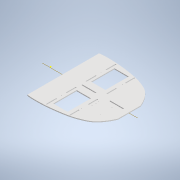
# Autodesk Inventor part: head_1
Saved by Autodesk Inventor 2020 (Build 240168000, 168)
## iProperties
Created: 2022-02-10
Part Number: head_1
Material: Типовые
Document SubType Name: Modeling
Designer: HP
Density: 1 g/cm^3
Appearance: По умолчанию
Mass: 318.083 g
Surface Area: 1630.63 cm^2
Volume: 318.083 cm^3
Author: HP
Autodesk Inventor part; units mm, degrees
ref_plane "YZ Plane" through (0, 0, 0) normal (1, 0, 0) x (0, 1, 0)
ref_plane "XZ Plane" through (0, 0, 0) normal (0, 1, 0) x (-1, 0, 0)
ref_plane "XY Plane" through (0, 0, 0) normal (0, 0, 1) x (1, 0, 0)
sketch "Эскиз1" plane through (0, 0, 0) normal (0, 1, 0) x (-1, 0, 0)
  line L0 (0, 0) -> (-339.5216, 0)
  line L1 (-129.0273, 2.0017) -> (-133.0273, 2.0017) construction
  line L2 (-133.0273, 20.9197) -> (-133.0273, 2.0017) construction
  line L3 (-133.0273, 20.9197) -> (-129.0273, 20.9197) construction
  line L4 (-129.0273, 20.9197) -> (-129.0273, 2.0017) construction
  line L5 (-129.0273, 2.0017) -> (-129.0273, -5.9794)
  line L6 (-10.1099, 0) -> (-40.1099, 0)
  line L7 (-53.7435, -154.1362) -> (-65.8717, -156.1972) construction
  line L8 (-65.8717, -156.1972) -> (-85.3727, -156.99) construction
  line L9 (-85.3727, -156.99) -> (-121.6794, -156.0387) construction
  line L10 (-121.6794, -156.0387) -> (-146.4123, -154.1362) construction
  line L11 (-146.4123, -154.1362) -> (-185.0972, -149.2213) construction
  line L12 (-185.0972, -149.2213) -> (-220.9282, -142.8795) construction
  line L13 (-220.9282, -142.8795) -> (-240.4292, -137.6475) construction
  line L14 (-240.4292, -137.6475) -> (-274.3577, -124.964) construction
  line L15 (-274.3577, -124.964) -> (-292.7488, -114.0244) construction
  line L16 (-292.7488, -114.0244) -> (-307.3349, -99.5969) construction
  line L17 (-307.3349, -99.5969) -> (-319.3843, -84.5352) construction
  line L18 (-319.3843, -84.5352) -> (-329.3726, -68.2051) construction
  line L19 (-329.3726, -68.2051) -> (-336.6657, -52.6677) construction
  line L20 (-336.6657, -52.6677) -> (-338.102, -47.8439) construction
  spline S0 degree 4 poles (-53.7435, -154.1362) (-65.8717, -156.1972) (-85.3727, -156.99) (-121.6794, -156.0387) (-146.4123, -154.1362) (-185.0972, -149.2213) (-220.9282, -142.8795) (-240.4292, -137.6475) (-274.3577, -124.964) (-292.7488, -114.0244) (-307.3349, -99.5969) (-319.3843, -84.5352) (-329.3726, -68.2051) (-336.6657, -52.6677) (-338.102, -47.8439) knots 1 1 1 1 1 2 3 4 5 6 7 8 9 10 11 12 12 12 12 12
  line L21 (-338.102, -47.8439) -> (-338.102, 0)
  line L22 (-53.7435, 154.1362) -> (-65.8717, 156.1972) construction
  line L23 (-65.8717, 156.1972) -> (-85.3727, 156.99) construction
  line L24 (-85.3727, 156.99) -> (-121.6794, 156.0387) construction
  line L25 (-121.6794, 156.0387) -> (-146.4123, 154.1362) construction
  line L26 (-146.4123, 154.1362) -> (-185.0972, 149.2213) construction
  line L27 (-185.0972, 149.2213) -> (-220.9282, 142.8795) construction
  line L28 (-220.9282, 142.8795) -> (-240.4292, 137.6475) construction
  line L29 (-240.4292, 137.6475) -> (-274.3577, 124.964) construction
  line L30 (-274.3577, 124.964) -> (-292.7488, 114.0244) construction
  line L31 (-292.7488, 114.0244) -> (-307.3349, 99.5969) construction
  line L32 (-307.3349, 99.5969) -> (-319.3843, 84.5352) construction
  line L33 (-319.3843, 84.5352) -> (-329.3726, 68.2051) construction
  line L34 (-329.3726, 68.2051) -> (-336.6657, 52.6677) construction
  line L35 (-336.6657, 52.6677) -> (-338.102, 47.8439) construction
  spline S1 degree 4 poles (-53.7435, 154.1362) (-65.8717, 156.1972) (-85.3727, 156.99) (-121.6794, 156.0387) (-146.4123, 154.1362) (-185.0972, 149.2213) (-220.9282, 142.8795) (-240.4292, 137.6475) (-274.3577, 124.964) (-292.7488, 114.0244) (-307.3349, 99.5969) (-319.3843, 84.5352) (-329.3726, 68.2051) (-336.6657, 52.6677) (-338.102, 47.8439) knots 1 1 1 1 1 2 3 4 5 6 7 8 9 10 11 12 12 12 12 12
  line L36 (-338.102, 47.8439) -> (-338.102, 0)
  line L37 (-144.7435, 0) -> (-53.7435, 0)
  line L38 (-53.7435, 0) -> (-53.7435, -154.1362)
  line L39 (-53.7435, 154.1362) -> (-65.8717, 156.1972) construction
  line L40 (-65.8717, 156.1972) -> (-85.3727, 156.99) construction
  line L41 (-85.3727, 156.99) -> (-121.6794, 156.0387) construction
  line L42 (-121.6794, 156.0387) -> (-146.4123, 154.1362) construction
  line L43 (-146.4123, 154.1362) -> (-185.0972, 149.2213) construction
  line L44 (-185.0972, 149.2213) -> (-220.9282, 142.8795) construction
  line L45 (-220.9282, 142.8795) -> (-240.4292, 137.6475) construction
  line L46 (-240.4292, 137.6475) -> (-274.3577, 124.964) construction
  line L47 (-274.3577, 124.964) -> (-292.7488, 114.0244) construction
  line L48 (-292.7488, 114.0244) -> (-307.3349, 99.5969) construction
  line L49 (-307.3349, 99.5969) -> (-319.3843, 84.5352) construction
  line L50 (-319.3843, 84.5352) -> (-329.3726, 68.2051) construction
  line L51 (-329.3726, 68.2051) -> (-336.6657, 52.6677) construction
  line L52 (-336.6657, 52.6677) -> (-338.102, 47.8439) construction
  spline S2 degree 4 poles (-53.7435, 154.1362) (-65.8717, 156.1972) (-85.3727, 156.99) (-121.6794, 156.0387) (-146.4123, 154.1362) (-185.0972, 149.2213) (-220.9282, 142.8795) (-240.4292, 137.6475) (-274.3577, 124.964) (-292.7488, 114.0244) (-307.3349, 99.5969) (-319.3843, 84.5352) (-329.3726, 68.2051) (-336.6657, 52.6677) (-338.102, 47.8439) knots 1 1 1 1 1 2 3 4 5 6 7 8 9 10 11 12 12 12 12 12
  line L53 (-338.102, 47.8439) -> (-338.102, 0)
  line L54 (-53.7435, 0) -> (-53.7435, 154.1362)
  point P0 (-144.7435, 57.7778)
  dimension "d42" = 30
  constraints: 18 end point, 15 symmetric about line, 5 point on line, 2 perpendicular, 1 horizontal, 1 vertical, 9 other
  measures "d42" distance of L6.start L6.end
extrude "Выдавливание1" add sketch "Эскиз1" along normal blind 4
sketch "Эскиз2" plane through (0, 0, 0) normal (0, -1, 0) x (1, 0, 0)
  line L0 (224, 59.917) -> (220, 59.917) projected
  line L1 (220, 59.917) -> (220, 19.9723) projected
  line L2 (220, 19.9723) -> (224, 19.9723) projected
  line L3 (224, 19.9723) -> (224, 59.917) projected
  line L4 (220, 99.8616) -> (224, 99.8616) projected
  line L5 (224, 99.8616) -> (224, 139.8063) projected
  line L6 (224, 139.8063) -> (220, 139.8063) projected
  line L7 (220, 139.8063) -> (220, 99.8616) projected
  line L8 (224, -19.9723) -> (220, -19.9723) projected
  line L9 (220, -19.9723) -> (220, -59.917) projected
  line L10 (220, -59.917) -> (224, -59.917) projected
  line L11 (224, -59.917) -> (224, -19.9723) projected
  line L12 (224, -99.8616) -> (220, -99.8616) projected
  line L13 (220, -99.8616) -> (220, -139.8063) projected
  line L14 (220, -139.8063) -> (224, -139.8063) projected
  line L15 (224, -139.8063) -> (224, -99.8616) projected
  line L16 (220, 19.9723) -> (219.5, 19.9723)
  line L17 (219.5, 19.9723) -> (219.5, 59.917)
  line L18 (219.5, 59.917) -> (220, 59.917)
  line L19 (224, 59.917) -> (224.5, 59.917)
  line L20 (224.5, 59.917) -> (224.5, 19.9723)
  line L21 (224.5, 19.9723) -> (224, 19.9723)
  line L22 (220, 99.8616) -> (219.5, 99.8616)
  line L23 (219.5, 99.8616) -> (219.5, 139.8063)
  line L24 (219.5, 139.8063) -> (220, 139.8063)
  line L25 (224, 99.8616) -> (224.5, 99.8616)
  line L26 (224.5, 99.8616) -> (224.5, 139.8063)
  line L27 (224.5, 139.8063) -> (224, 139.8063)
  line L28 (197.5179, 0) -> (240.56, 0)
  line L29 (224, -59.917) -> (220, -59.917)
  line L30 (220, -59.917) -> (220, -19.9723)
  line L31 (220, -19.9723) -> (224, -19.9723)
  line L32 (224, -19.9723) -> (224, -59.917)
  line L33 (220, -99.8616) -> (224, -99.8616)
  line L34 (224, -99.8616) -> (224, -139.8063)
  line L35 (224, -139.8063) -> (220, -139.8063)
  line L36 (220, -139.8063) -> (220, -99.8616)
  line L37 (220, -19.9723) -> (219.5, -19.9723)
  line L38 (219.5, -19.9723) -> (219.5, -59.917)
  line L39 (219.5, -59.917) -> (220, -59.917)
  line L40 (224, -59.917) -> (224.5, -59.917)
  line L41 (224.5, -59.917) -> (224.5, -19.9723)
  line L42 (224.5, -19.9723) -> (224, -19.9723)
  line L43 (220, -99.8616) -> (219.5, -99.8616)
  line L44 (219.5, -99.8616) -> (219.5, -139.8063)
  line L45 (219.5, -139.8063) -> (220, -139.8063)
  line L46 (224, -99.8616) -> (224.5, -99.8616)
  line L47 (224.5, -99.8616) -> (224.5, -139.8063)
  line L48 (224.5, -139.8063) -> (224, -139.8063)
  point P0 (0, 0)
  dimension "d67" = 4
  dimension "d68" = 0.5
  dimension "d69" = 0.5
  dimension "d70" = 0.5
  dimension "d71" = 0.5
  constraints: 66 end point, 8 symmetric about line, 6 perpendicular, 4 horizontal, 4 point on line, 2 parallel
  measures "d67" distance between parallel lines of L3 L1
  measures "d68" distance of L1.end L16.end
  measures "d69" distance of L0.start L19.end
  measures "d70" distance of L4.start L22.end
  measures "d71" distance of L4.end L25.end
extrude "Выдавливание2" cut sketch "Эскиз2" against normal blind 4
sketch "Эскиз3" plane through (0, 0, 0) normal (0, -1, 0) x (1, 0, 0)
  line L0 (129.0273, -150.1475) -> (133.0273, -150.1475) projected
  line L1 (133.0273, -150.1475) -> (133.0273, -107.3807) projected
  line L2 (133.0273, -107.3807) -> (129.0273, -107.3807) projected
  line L3 (129.0273, -107.3807) -> (129.0273, -150.1475) projected
  line L4 (133.0273, -64.6139) -> (133.0273, -21.8471) projected
  line L5 (133.0273, -21.8471) -> (129.0273, -21.8471) projected
  line L6 (129.0273, -21.8471) -> (129.0273, -64.6139) projected
  line L7 (129.0273, -64.6139) -> (133.0273, -64.6139) projected
  line L8 (129.0273, 63.6865) -> (129.0273, 20.9197) projected
  line L9 (133.0273, 20.9197) -> (133.0273, 63.6865) projected
  line L10 (133.0273, 63.6865) -> (129.0273, 63.6865) projected
  line L11 (129.0273, 63.6865) -> (129.0273, 20.9197) projected
  line L12 (129.0273, 20.9197) -> (133.0273, 20.9197) projected
  line L13 (129.0273, 149.2201) -> (129.0273, 106.4533) projected
  line L14 (129.0273, 106.4533) -> (133.0273, 106.4533) projected
  line L15 (133.0273, 106.4533) -> (133.0273, 149.2201) projected
  line L16 (133.0273, 149.2201) -> (129.0273, 149.2201) projected
  line L17 (129.0273, 149.2201) -> (129.0273, 106.4533) projected
  line L18 (129.0273, 20.9197) -> (128.5273, 20.9197)
  line L19 (128.5273, 20.9197) -> (128.5273, 63.6865)
  line L20 (128.5273, 63.6865) -> (129.0273, 63.6865)
  line L21 (133.0273, 63.6865) -> (133.5273, 63.6865)
  line L22 (133.5273, 63.6865) -> (133.5273, 20.9197)
  line L23 (133.5273, 20.9197) -> (133.0273, 20.9197)
  line L24 (129.0273, 106.4533) -> (128.5273, 106.4533)
  line L25 (128.5273, 106.4533) -> (128.5273, 149.2201)
  line L26 (128.5273, 149.2201) -> (129.0273, 149.2201)
  line L27 (133.0273, 149.2201) -> (133.5273, 149.2201)
  line L28 (133.5273, 149.2201) -> (133.5273, 106.4533)
  line L29 (133.0273, 106.4533) -> (133.5273, 106.4533)
  line L30 (121.8366, 0) -> (139.2752, 0)
  line L31 (129.0273, -150.1475) -> (128.5273, -150.1475)
  line L32 (128.5273, -150.1475) -> (128.5273, -107.3807)
  line L33 (128.5273, -107.3807) -> (129.0273, -107.3807)
  line L34 (133.0273, -107.3807) -> (132.5273, -107.3807)
  line L35 (132.5273, -107.3807) -> (132.5273, -150.1475)
  line L36 (132.5273, -150.1475) -> (133.0273, -150.1475)
  line L37 (129.0273, -64.6139) -> (128.5273, -64.6139)
  line L38 (128.5273, -64.6139) -> (128.5273, -21.8471)
  line L39 (128.5273, -21.8471) -> (129.0273, -21.8471)
  line L40 (133.0273, -21.8471) -> (132.5273, -21.8471)
  line L41 (132.5273, -21.8471) -> (132.5273, -64.6139)
  line L42 (133.0273, -64.6139) -> (132.5273, -64.6139)
  point P0 (0, 0)
  dimension "d72" = 0.5
  dimension "d73" = 0.5
  dimension "d74" = 0.5
  constraints: 50 end point, 16 point on line, 9 perpendicular, 3 horizontal, 2 parallel, 1 collinear
  measures "d72" distance of L8.end L18.end
  measures "d73" distance of L9.end L21.end
  measures "d74" distance of L13.end L24.end
extrude "Выдавливание3" cut sketch "Эскиз3" against normal blind 4
sketch "Эскиз6" plane through (0, 0, 0) normal (0, -1, 0) x (1, 0, 0)
  line L0 (74.396, 0) -> (255.7791, 0)
  line L1 (174.802, 33.2852) -> (169.6077, 33.2852) projected
  line L2 (180.6651, 129.1508) -> (169.6077, 129.1508) projected
  line L3 (145.3577, 104.101) -> (145.3577, 81.101) projected
  line L4 (142.5064, 31.2611) -> (204.162, 31.2611)
  line L5 (204.162, 31.2611) -> (204.162, 131.4427)
  line L6 (204.162, 131.4427) -> (142.5064, 131.4427)
  line L7 (142.5064, 131.4427) -> (142.5064, 31.2611)
  line L8 (174.802, -33.2852) -> (169.6077, -33.2852)
  line L9 (180.6651, -129.1508) -> (169.6077, -129.1508)
  line L10 (145.3577, -104.101) -> (145.3577, -81.101)
  line L11 (142.5064, -31.2611) -> (204.162, -31.2611)
  line L12 (204.162, -31.2611) -> (204.162, -131.4427)
  line L13 (204.162, -131.4427) -> (142.5064, -131.4427)
  line L14 (142.5064, -131.4427) -> (142.5064, -31.2611)
  point P0 (0, 0)
  constraints: 24 end point, 10 symmetric about line, 2 horizontal, 2 parallel, 1 perpendicular
sketch "Эскиз7" plane through (0, 0, 0) normal (0, -1, 0) x (1, 0, 0)
  line L0 (193.6883, 2) -> (133.9866, 2) projected
  line L1 (133.9866, -2) -> (193.6883, -2) projected
  line L2 (193.6883, -2) -> (193.6883, 2) projected
  line L3 (193.6883, 2) -> (133.9866, 2) projected
  line L4 (133.9866, 2) -> (133.9866, -2) projected
  line L5 (313.0917, 2) -> (253.39, 2) projected
  line L6 (253.39, -2) -> (313.0917, -2) projected
  line L7 (133.9866, 2) -> (133.9866, -2) projected
  line L8 (133.9866, -2) -> (193.6883, -2) projected
  line L9 (193.6883, -2) -> (193.6883, 2) projected
  line L10 (133.9866, 2) -> (133.9866, 2.5)
  line L11 (133.9866, 2.5) -> (193.6883, 2.5)
  line L12 (193.6883, 2.5) -> (193.6883, 2)
  line L13 (193.6883, -2) -> (193.6883, -2.5)
  line L14 (193.6883, -2.5) -> (133.9866, -2.5)
  line L15 (133.9866, -2.5) -> (133.9866, -2)
  line L16 (253.39, 2) -> (253.39, -2) projected
  line L17 (313.0917, -2) -> (313.0917, 2) projected
  point P0 (0, 0)
  point P1 (193.6883, -1.5)
  dimension "d75" = 0.5
  dimension "d76" = 0.5
  constraints: 12 end point, 5 perpendicular, 2 point on line
  measures "d75" distance of L0.end L10.end
  measures "d76" distance of L8.end L13.end
extrude "Выдавливание7" cut sketch "Эскиз7" against normal through all contours L2 L1 L4 L0 | L0 L10 L11 L12 | L13 L14 L15 L1
sketch "Эскиз8" plane through (0, 0, 0) normal (0, -1, 0) x (1, 0, 0)
  line L0 (133.0273, 82.3199) -> (133.0273, 83.6199) projected
  line L1 (129.0273, 82.3199) -> (133.0273, 82.3199) projected
  line L2 (129.0273, 83.6199) -> (129.0273, 82.3199) projected
  line L3 (129.0273, 83.6199) -> (133.0273, 83.6199) projected
  line L4 (133.0273, 86.5199) -> (133.0273, 87.8199) projected
  line L5 (129.0273, 86.5199) -> (133.0273, 86.5199) projected
  line L6 (129.0273, 87.8199) -> (129.0273, 86.5199) projected
  line L7 (129.0273, 87.8199) -> (133.0273, 87.8199) projected
  line L8 (129.0273, 83.6199) -> (133.0273, 83.6199)
  line L9 (133.0273, 83.6199) -> (133.0273, 86.5199)
  line L10 (133.0273, 86.5199) -> (129.0273, 86.5199)
  line L11 (129.0273, 86.5199) -> (129.0273, 83.6199)
  circle A0 centre (130.4773, 85.0699) radius 1.45
  line L12 (129.0273, 0) -> (153.0576, 0)
  line L13 (129.0273, -87.4491) -> (132.0273, -87.4491)
  line L14 (132.0273, -87.4491) -> (132.0273, -84.5491)
  line L15 (132.0273, -84.5491) -> (129.0273, -84.5491)
  line L16 (129.0273, -84.5491) -> (129.0273, -87.4491)
  circle A1 centre (130.4773, -85.9991) radius 1.45
  point P0 (0, 0)
  dimension "d44" = 3
  dimension "d45" = 2.9
  constraints: 18 end point, 6 tangent, 4 parallel, 3 horizontal, 2 centre point, 2 perpendicular
  measures "d44" distance of L15.end L14.end
  measures "d45" distance of L14.end L13.end
extrude "Выдавливание8" cut sketch "Эскиз8" against normal through all contours A0 | A1
sketch "Эскиз9" plane through (0, 0, 0) normal (0, -1, 0) x (1, 0, 0)
  line L0 (253.39, -1.5) -> (313.0917, -1.5) projected
  line L1 (313.0917, 1.5) -> (253.39, 1.5) projected
  line L2 (313.0917, -1.5) -> (313.0917, 1.5) projected
  line L3 (253.39, 1.5) -> (253.39, -1.5) projected
  line L4 (253.39, 1.5) -> (253.39, 2)
  line L5 (253.39, 2) -> (313.0917, 2)
  line L6 (313.0917, 2) -> (313.0917, 1.5)
  line L7 (313.0917, -1.5) -> (313.0917, -2)
  line L8 (313.0917, -2) -> (253.39, -2)
  line L9 (253.39, -2) -> (253.39, -1.5)
  point P0 (0, 0)
  dimension "d77" = 0.5
  dimension "d78" = 0.5
  constraints: 12 end point, 4 perpendicular, 2 point on line, 1 parallel
  measures "d77" distance of L1.end L4.end
  measures "d78" distance of L0.end L7.end
extrude "Выдавливание9" cut sketch "Эскиз9" against normal through all
extrude "Выдавливание10" cut sketch "Эскиз6" against normal through all
sketch "Эскиз10" plane through (0, 0, 0) normal (0, -1, 0) x (1, 0, 0)
  line L0 (220, 89.4199) -> (223, 89.4199) projected
  line L1 (223, 86.5199) -> (220, 86.5199) projected
  line L2 (223, 86.5199) -> (223, 89.4199)
  circle A0 centre (221.55, 87.9699) radius 1.45
  line L3 (223, 0) -> (202.3456, 0)
  circle A1 centre (221.55, -87.9699) radius 1.45
  point P0 (0, 0)
  dimension "d52" = 2.9
  constraints: 4 end point, 3 tangent, 2 centre point, 1 horizontal, 1 symmetric about line, 1 vertical, 1 other
  measures "d52" diameter of A0
extrude "Выдавливание11" cut sketch "Эскиз10" against normal through all contours A0 | A1
sketch "Эскиз11" plane through (0, 4, 0) normal (0, 1, 0) x (1, 0, 0)
  point P0 (0, 0)
sketch "Эскиз12" plane through (0, 0, 0) normal (0, -1, 0) x (1, 0, 0)
  line L0 (223, 19.9723) -> (223, 59.917) projected
  line L1 (223, 19.9723) -> (232.5, 19.9723)
  line L2 (223, 59.917) -> (223, 19.9723) projected
  line L3 (232.5, 139.4752) -> (232.5, 54.4752)
  circle A0 centre (232.5, 54.4752) radius 0.05
  point P0 (0, 0)
  point P1 (53.7435, 154.1362)
  point P2 (338.102, 47.8439)
  dimension "d55" = 9.5
  dimension "d56" = 85
  dimension "d60" = 0.1
  constraints: 4 end point, 2 coincident, 1 centre point, 1 horizontal, 1 vertical, 2 other
  measures "d55" distance of L0.start L1.end
  measures "d56" distance of L3.start L3.end
  measures "d60" diameter of A0
extrude "Выдавливание12" cut sketch "Эскиз12" against normal blind 0.1
sketch "Эскиз13" plane through (0, 4, 0) normal (0, 1, 0) x (1, 0, 0)
  ellipse E0 centre (232.5, -54.5049) end of major axis (231.7, -54.5039) minor radius 0.7999
  line L0 (232.4894, -27.3693) -> (232.4888, -25.7695)
  line L1 (233.2891, -26.566) -> (231.6891, -26.5666)
  line L2 (284.8274, -22.2697) -> (284.8268, -20.67)
  line L3 (282.5059, -69.7229) -> (284.1059, -69.7223)
  line L4 (283.3059, -69.7226) -> (283.3056, -68.9228)
  line L5 (283.3059, -69.7226) -> (283.3062, -70.5225)
  circle A0 centre (283.3059, -69.7226) radius 1.45
  circle A1 centre (284.8271, -21.4699) radius 1.45
  circle A2 centre (232.4891, -26.5663) radius 1.45
  circle A3 centre (232.5, -54.5049) radius 1.45
  point P0 (0, 0)
extrude "Выдавливание13" cut sketch "Эскиз13" against normal through all contours E0 | A0 | A1 | A2 | A3
sketch "Эскиз14" plane through (0, 0, 0) normal (0, -1, 0) x (1, 0, 0)
  circle A0 centre (232.4891, 26.5663) radius 1.45 projected
  circle A1 centre (232.5, 54.5049) radius 1.45 projected
  line L0 (232.4891, 26.5663) -> (232.5, 54.5049)
  line L1 (232.4945, 40.5356) -> (232.4937, 38.3996)
  circle A2 centre (232.4937, 38.3996) radius 1.5
  point P0 (0, 0)
  dimension "d82" = 2.136
  dimension "d83" = 3
  constraints: 4 end point, 1 centre point, 1 coincident, 1 midpoint, 1 point on line
  measures "d82" distance of L1.start L1.end
  measures "d83" diameter of A2
extrude "Выдавливание14" cut sketch "Эскиз14" against normal through all contours A2 L0 | L0 A2
sketch "Эскиз15" plane through (0, 0, 0) normal (0, -1, 0) x (1, 0, 0)
  circle A0 centre (232.4937, 38.3996) radius 1.5 projected
  circle A1 centre (232.4937, 11.5105) radius 1.5 projected
  circle A2 centre (232.4937, -11.5113) radius 1.5 projected
  circle A3 centre (232.4937, -38.4004) radius 1.5 projected
  circle A4 centre (299.5428, 38.3996) radius 1.5 projected
  circle A5 centre (299.5428, 22.8428) radius 1.5 projected
  circle A6 centre (299.5428, -22.8436) radius 1.5 projected
  circle A7 centre (299.5428, -38.4004) radius 1.5 projected
  point P0 (0, 0)
extrude "Выдавливание15" cut sketch "Эскиз15" against normal through all
